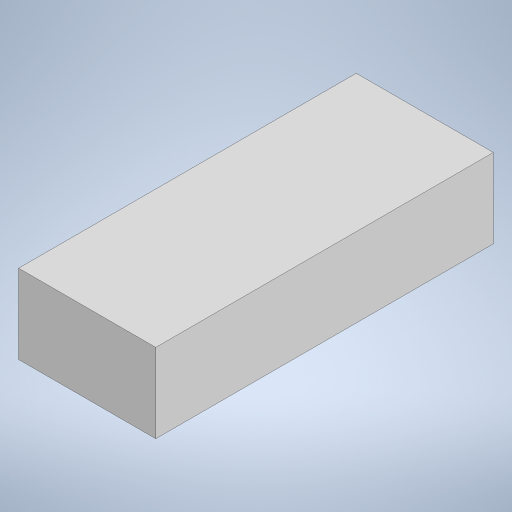
# Autodesk Inventor part: RectOuterEye
Saved by Autodesk Inventor 2024.3 (Build 283343000, 343)
## iProperties
Created: 2024-06-20
Part Number: RectOuterEye
Material: 一般
Document SubType Name: Modeling
Designer: yukin
Density: 1 g/cm^3
Appearance: 既定
Author: yukin
Autodesk Inventor part; units mm, degrees
ref_plane "YZ Plane" through (0, 0, 0) normal (1, 0, 0) x (0, 1, 0)
ref_plane "XZ Plane" through (0, 0, 0) normal (0, 1, 0) x (-1, 0, 0)
ref_plane "XY Plane" through (0, 0, 0) normal (0, 0, 1) x (1, 0, 0)
sketch "スケッチ1" plane through (0, 0, 0) normal (0, 1, 0) x (-1, 0, 0)
  line L0 (1.1468, 2.3153) -> (-1.4532, 2.3153)
  line L1 (-1.4532, 2.3153) -> (-1.4532, -4.0847)
  line L2 (-1.4532, -4.0847) -> (1.1468, -4.0847)
  line L3 (1.1468, -4.0847) -> (1.1468, 2.3153)
  point P0 (0, 0)
  dimension "d0" = 2.6
  dimension "d1" = 6.4
  constraints: 8 end point, 2 parallel, 1 horizontal, 1 perpendicular
  measures "d0" distance of L0.start L0.end
  measures "d1" distance of L2.end L0.start
extrude "押し出し1" add sketch "スケッチ1" along normal blind 1.5
